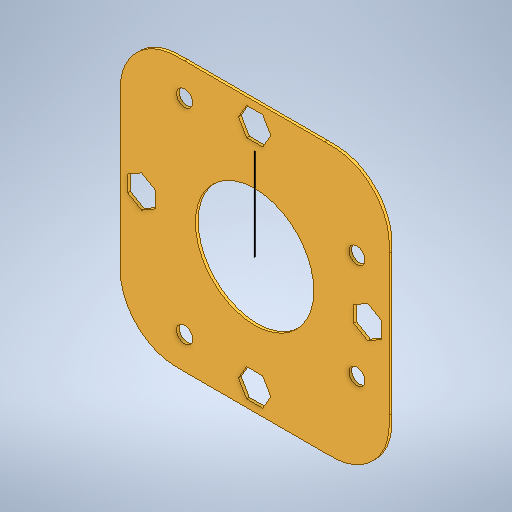
# Autodesk Inventor part: CONECTOR DE ACOPLE A AVION test
Saved by Autodesk Inventor 2025.3 (Build 293356030, 356C)
## iProperties
Created: 2025-07-11
Part Number: CONECTOR DE ACOPLE A AVION test
Material: Generic
Document SubType Name: Modeling
Designer: jv
Density: 1 g/cm^3
Appearance: Default(1)
Author: jv
Autodesk Inventor part; units mm, degrees
ref_plane "YZ Plane" through (0, 0, 0) normal (1, 0, 0) x (0, 1, 0)
ref_plane "XZ Plane" through (0, 0, 0) normal (0, 1, 0) x (-1, 0, 0)
ref_plane "XY Plane" through (0, 0, 0) normal (0, 0, 1) x (1, 0, 0)
sketch "Sketch1" plane through (0, 0, 0) normal (0, 0, 1) x (1, 0, 0)
  line L0 (-25, 25) -> (25, 25)
  line L1 (25, 25) -> (25, -25)
  line L2 (25, -25) -> (-25, -25)
  line L3 (-25, -25) -> (-25, 25)
  circle A0 centre (0, 0) radius 11
  circle A1 centre (-13, 19) radius 1.5
  circle A2 centre (19, 9.75) radius 1.5
  line L4 (19, 0) -> (19, 9.75)
  line L5 (-53.0419, 0) -> (53.0419, 0)
  circle A3 centre (19, -9.75) radius 1.5
  circle A4 centre (-13, -19) radius 1.5
  line L6 (19, 11.25) -> (-4.8981, 11.25)
  point P0 (0, 25)
  point P1 (25, 0)
  point P2 (25, 9.75)
  point P3 (20.5, 9.75)
  point P4 (-11.5, 19)
  point P5 (19, -11.25)
  point P6 (-13, 20.5)
  point P7 (-13, -20.5)
  point P8 (11, 0)
  point P9 (11, 0)
  point P10 (-11, 0)
  dimension "d49" = 3
  dimension "d56" = 30.3101
  dimension "d0" = 50
  dimension "d1" = 22
  dimension "d2" = 50
  dimension "d3" = 3
  dimension "d6" = 3
  dimension "d10" = 19.5
  dimension "d11" = 13
  dimension "d12" = 19
  dimension "d46" = 12
  dimension "d48" = 8.8556
  dimension "d50" = 8.8556
  dimension "d52" = 35
  dimension "d53" = 38
  dimension "d54" = 16.5
  dimension "d55" = 10.5217
  dimension "d61" = 36.5
  dimension "d62" = 22.5
  dimension "d63" = 41
  dimension "d64" = 4.5
  dimension "d112" = 14
  dimension "d113" = 14
  dimension "d114" = 12
  dimension "d115" = 6
  dimension "d117" = 13
  dimension "d118" = 40.0182
  constraints: 14 end point, 7 vertical alignment, 6 point on circle, 4 horizontal alignment, 3 centre point, 3 coincident, 3 horizontal, 3 midpoint, 3 point on line, 2 parallel, 2 symmetric about line, 1 perpendicular, 1 vertical, 6 other
  measures "d0" distance of L0.start L0.end
  measures "d1" diameter of A0
  measures "d2" distance of L2.end L0.start
  measures "d3" diameter of A1
  measures "d6" diameter of A2
  measures "d10" diameter of L4.end L5
  measures "d11" horizontal distance of point (0, 0) A1.centre
  measures "d12" horizontal distance of point (0, 0) L4.end
  measures "d46" distance from line of L3 A1.centre
  measures "d53" distance of point (-13, -19) A1.centre
  measures "d61" distance from line of L1 A1.start
  measures "d62" distance of L6.start point (19, -11.25)
  measures "d63" distance of A1.end point (-13, -20.5)
  measures "d64" distance from line of L1 A2.start
  measures "d112" distance from line of L1 point (11, 0)
  measures "d113" distance from line of L3 A0.end
  measures "d114" distance from line of L3 point (-13, -19)
  measures "d115" distance from line of L1 point (19, -9.75)
  measures "d117" horizontal distance of point (0, 0) point (-13, -19)
extrude "Extrusion1" add sketch "Sketch1" along normal blind 0.5 contours L0 L1 L5 A0 L3 | L5 A0 L1 L2 L3
sketch "Sketch3" plane through (0, 0, 0.5) normal (0, 0, 1) x (1, 0, 0)
  line L0 (-4, 25) -> (4, 25)
  line L1 (4, 25) -> (4, -25)
  line L2 (4, -25) -> (-4, -25)
  line L3 (-4, -25) -> (-4, 25)
  circle A0 centre (12.5, 0) radius 2
  circle A1 centre (-12.5, 0) radius 2
  circle A2 centre (21, 0) radius 1.6
  circle A3 centre (0, 21) radius 1.6
  circle A4 centre (-21, 0) radius 1.6
  circle A5 centre (0, -21) radius 1.6
  line L4 (-25, -4) -> (-25, 4)
  line L5 (-25, 4) -> (25, 4)
  line L6 (25, -4) -> (-25, -4)
  line L7 (25, 4) -> (25, -4)
  circle A6 centre (0, 21) radius 4
  circle A7 centre (21, 0) radius 4
  circle A8 centre (-21, 0) radius 4
  circle A9 centre (0, -21) radius 4
  circle A10 centre (12.5, 12.5) radius 8.5
  circle A11 centre (-12.5, 12.5) radius 8.5
  circle A12 centre (-12.5, -12.5) radius 8.5
  circle A13 centre (12.5, -12.5) radius 8.5
  circle A14 centre (0, 0) radius 4
  circle A15 centre (0, 9.5) radius 2
  circle A16 centre (0, -9.5) radius 2
  point P0 (4, 0)
  point P1 (0, 25)
  point P2 (-25, 0)
  point P3 (0, 4)
  dimension "d75" = 4
  dimension "d76" = 360
  dimension "d77" = 3.2
  dimension "d78" = 360
  dimension "d79" = 8
  dimension "d80" = 90
  dimension "d81" = 50
  dimension "d82" = 42
  dimension "d83" = 4
  dimension "d84" = 17
  dimension "d85" = 360
  dimension "d86" = 4
  dimension "d87" = 360
  dimension "d88" = 19
  dimension "d89" = 25
  constraints: 16 end point, 14 centre point, 6 coincident, 3 horizontal alignment, 2 midpoint, 2 parallel, 2 tangent, 2 vertical alignment, 1 horizontal, 1 perpendicular, 45 other
  measures "d75" diameter of A0
  measures "d77" diameter of A2
  measures "d79" distance of L1.end L3.start
  measures "d81" distance between parallel lines of L2 L0
  measures "d82" distance of A5.centre A3.centre
  measures "d83" distance of point (0, 25) point (0, 21)
  measures "d84" diameter of A10
  measures "d86" diameter of A15
  measures "d88" distance of A16.centre A15.centre
  measures "d89" distance of A0.centre A1.centre
extrude "Extrusion3" cut sketch "Sketch3" against normal blind 7 contours A2 | A3 | A4 | A5
fillet "Fillet1" radius 12 4 edges at (-25, 25, 0.25) (25, 25, 0.25) (25, -25, 0.25) (-25, -25, 0.25) curvature continuous yes
sketch "Sketch5" plane through (0, 0, 0) normal (0, 0, -1) x (-1, 0, 0)
  circle A0 centre (0, 21) radius 3
  circle A1 centre (0, 21) radius 1.5
  line L0 (1.5, 23.5981) -> (3, 21)
  line L1 (-1.5, 23.5981) -> (1.5, 23.5981)
  line L2 (-3, 21) -> (-1.5, 23.5981)
  line L3 (-1.5, 18.4019) -> (-3, 21)
  line L4 (1.5, 18.4019) -> (-1.5, 18.4019)
  line L5 (3, 21) -> (1.5, 18.4019)
  circle A2 centre (0, 21) radius 1.6 projected
  circle A3 centre (21, 0) radius 1.6 projected
  circle A4 centre (-21, 0) radius 1.6 projected
  circle A5 centre (0, -21) radius 1.6 projected
  circle A6 centre (-21, 0) radius 3
  circle A7 centre (-21, 0) radius 1.5
  line L6 (-23.5981, 1.5) -> (-21, 3)
  line L7 (-23.5981, -1.5) -> (-23.5981, 1.5)
  line L8 (-21, -3) -> (-23.5981, -1.5)
  line L9 (-18.4019, -1.5) -> (-21, -3)
  line L10 (-18.4019, 1.5) -> (-18.4019, -1.5)
  line L11 (-21, 3) -> (-18.4019, 1.5)
  circle A8 centre (0, -21) radius 3
  circle A9 centre (0, -21) radius 1.5
  line L12 (-1.5, -23.5981) -> (-3, -21)
  line L13 (1.5, -23.5981) -> (-1.5, -23.5981)
  line L14 (3, -21) -> (1.5, -23.5981)
  line L15 (1.5, -18.4019) -> (3, -21)
  line L16 (-1.5, -18.4019) -> (1.5, -18.4019)
  line L17 (-3, -21) -> (-1.5, -18.4019)
  circle A10 centre (21, 0) radius 3
  circle A11 centre (21, 0) radius 1.5
  line L18 (23.5981, -1.5) -> (21, -3)
  line L19 (23.5981, 1.5) -> (23.5981, -1.5)
  line L20 (21, 3) -> (23.5981, 1.5)
  line L21 (18.4019, 1.5) -> (21, 3)
  line L22 (18.4019, -1.5) -> (18.4019, 1.5)
  line L23 (21, -3) -> (18.4019, -1.5)
  line L24 (0, 0) -> (7.0109, 0)
  point P0 (-1.5, 23.5981)
  point P1 (-23.5981, -1.5)
  point P2 (1.5, -23.5981)
  point P3 (23.5981, 1.5)
  point P4 (-1.5, -18.4019)
  point P5 (-3, -21)
  point P6 (-1.5, -23.5981)
  point P7 (1.5, -23.5981)
  point P8 (3, -21)
  point P9 (1.5, -18.4019)
  point P10 (18.4019, -1.5)
  point P11 (21, -3)
  point P12 (23.5981, -1.5)
  point P13 (23.5981, 1.5)
  point P14 (21, 3)
  point P15 (18.4019, 1.5)
  point P16 (1.5, 18.4019)
  point P17 (3, 21)
  point P18 (1.5, 23.5981)
  point P19 (-1.5, 23.5981)
  point P20 (-3, 21)
  point P21 (-1.5, 18.4019)
  point P22 (-18.4019, 1.5)
  point P23 (-21, 3)
  point P24 (-23.5981, 1.5)
  point P25 (-23.5981, -1.5)
  point P26 (-21, -3)
  point P27 (-18.4019, -1.5)
  dimension "d96" = 6
  dimension "d97" = 3
  dimension "d100" = 360
  dimension "d104" = 360
  dimension "d108" = 360
  constraints: 50 end point, 5 coincident, 4 centre point, 1 horizontal, 1 parallel, 143 other
  measures "d97" diameter of A1
extrude "Extrusion4" cut sketch "Sketch5" against normal blind 2.1 contours L5 L4 L3 L2 L1 L0 | L10 L9 L8 L7 L6 L11 | L14 L13 L12 L17 L16 L15 | L19 L18 L23 L22 L21 L20
sketch "Sketch6" plane through (0, 0, 0.5) normal (0, 0, 1) x (1, 0, 0)
  line L0 (0, 0) -> (0, 16.9544)
  constraints: 2 end point, 1 vertical
body "Solid1"
